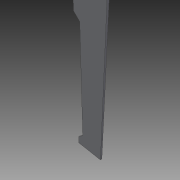
# Autodesk Inventor part: inner_brace_right
Saved by Autodesk Inventor 2014 (Build 180170000, 170)
## iProperties
Created: 2014-03-31
Part Number: inner_brace_right
Material: Generic
Document SubType Name: Modeling
Designer: buben
Density: 1 g/cm^3
Appearance: Default
Author: buben
Autodesk Inventor part; units mm, degrees
ref_plane "YZ Plane" through (0, 0, 0) normal (1, 0, 0) x (0, 1, 0)
ref_plane "XZ Plane" through (0, 0, 0) normal (0, 1, 0) x (-1, 0, 0)
ref_plane "XY Plane" through (0, 0, 0) normal (0, 0, 1) x (1, 0, 0)
sketch "Sketch1" plane through (0, 0, 0) normal (0, 1, 0) x (-1, 0, 0)
  line L0 (0, 0) -> (-100, 0)
  line L1 (-100, 0) -> (-100, -489)
  line L2 (-100, -489) -> (0, -489)
  line L3 (0, -489) -> (0, 0)
  dimension "d0" = 489
  dimension "d1" = 100
  constraints: 8 end point, 2 parallel, 1 horizontal, 1 perpendicular
  measures "d0" distance of L2.end L0.start
  measures "d1" distance of L0.start L0.end
extrude "Extrusion1" add sketch "Sketch1" along normal blind 6.5
sketch "Sketch2" plane through (0, 6.5, 0) normal (0, 1, 0) x (1, 0, 0)
  line L0 (0, 489) -> (0, 0) projected
  line L1 (0, 459) -> (20, 439)
  line L2 (20, 439) -> (20, 65)
  line L3 (20, 65) -> (0, 45)
  line L4 (0, 459) -> (0, 45)
  dimension "d4" = 45
  dimension "d5" = 20
  dimension "d6" = 30
  dimension "d7" = 45
  constraints: 8 end point, 2 parallel, 2 point on line, 1 perpendicular
  measures "d4" angle of L0 L1
  measures "d5" distance between parallel lines of L0 L2
  measures "d6" distance of L0.start L1.start
  measures "d7" distance of L0.end L3.end
extrude "Extrusion2" cut sketch "Sketch2" against normal through all
body "Solid1"
